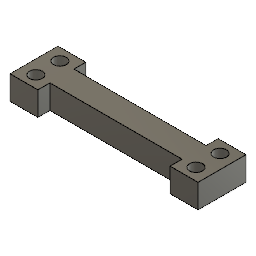
enclosure v64 (Autodesk Fusion 360 archive; units mm, degrees)
design "Load Cell"
Autodesk Fusion 360 part; units mm, degrees
sketch "Sketch1" plane through (0, 0, 0) normal (0, 1, 0) x (1, 0, 0)
  circle A0 centre (0, 0) radius 1.6
  line L0 (0, 0) -> (0, -6) construction
  circle A1 centre (0, -6) radius 1.6
  line L1 (0, -3) -> (40, -3) construction
  line L2 (-3.5, 3) -> (3.5, 3)
  line L3 (3.5, 3) -> (3.5, -9)
  line L4 (3.5, -9) -> (-3.5, -9)
  line L5 (-3.5, -9) -> (-3.5, 3)
  line L6 (20, -3) -> (20, -8.5486) construction
  circle A2 centre (40, 0) radius 1.6
  circle A3 centre (40, -6) radius 1.6
  line L7 (40, 0) -> (40, -6) construction
  line L8 (36.5, 3) -> (36.5, -9)
  line L9 (36.5, -9) -> (43.5, -9)
  line L10 (43.5, -9) -> (43.5, 3)
  line L11 (43.5, 3) -> (36.5, 3)
  line L12 (3.5, -0.0084) -> (36.5, -0.0084)
  line L13 (36.5, -0.0084) -> (36.5, -5.9916)
  line L14 (36.5, -5.9916) -> (3.5, -5.9916)
  line L15 (3.5, -5.9916) -> (3.5, -0.0084)
  point P0 (40, 0)
  point P1 (40, -3)
  dimension "d1" = 3.2
  dimension "d2" = 6
  dimension "d3" = 3.2
  dimension "d5" = 40
  dimension "d6" = 7
  dimension "d7" = 12
  constraint coincident A0.centre L0.start
  constraint vertical L0
  constraint coincident L0.end A1.centre
  constraint midpoint L0 L1.start
  constraint perpendicular L0 L1
  constraint horizontal L2
  constraint vertical L3
  constraint horizontal L4
  constraint vertical L5
  constraint symmetric L0 L3 L5
  constraint symmetric L1 L2 L4
  constraint midpoint L1 L6.start
  constraint perpendicular L1 L6
  constraint symmetric A0.centre L6 A2.centre
  constraint symmetric A0 L6 A2
  constraint symmetric A0.centre L6 P0
  constraint symmetric L0.end L6 A3.centre
  constraint symmetric A1 L6 A3
  constraint symmetric L1.start L6 P1
  constraint symmetric L2.start L6 L10.end
  constraint symmetric L2.end L6 L8.start
  constraint symmetric L3.end L6 L8.end
  constraint symmetric L4.end L6 L9.end
  constraint horizontal L12
  constraint vertical L13
  constraint horizontal L14
  constraint vertical L15
  constraint coincident L8 L13.end
  constraint coincident L3 L12.start
  constraint symmetric L1 L12 L14
  measures "d1" diameter of A0
  measures "d2" distance of A0.centre L0.end
  measures "d3" diameter of A1
  measures "d5" distance of L0 P1
  measures "d6" distance of L2.start L2.end
  measures "d7" distance of L2.start L4.end
extrude "Extrude1" add sketch "Sketch1" along normal blind 6

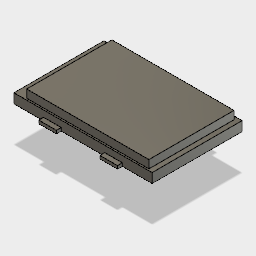
design "Display"
Autodesk Fusion 360 part; units mm, degrees
sketch "Sketch1" plane through (0, 0, 0) normal (0, 1, 0) x (1, 0, 0)
  line L0 (0, 0) -> (86, 0)
  line L1 (86, 0) -> (86, -56)
  line L2 (86, -56) -> (0, -56)
  line L3 (0, -56) -> (0, 0)
  line L4 (7, -2) -> (83, -2)
  line L5 (83, -2) -> (83, -55)
  line L6 (83, -55) -> (7, -55)
  line L7 (7, -55) -> (7, -2)
  line L8 (18.5, 3) -> (29.5, 3)
  line L9 (29.5, 3) -> (29.5, -59)
  line L10 (29.5, -59) -> (18.5, -59)
  line L11 (18.5, -59) -> (18.5, 3)
  line L12 (43, 0) -> (43, -72.5611) construction
  line L13 (86, -28) -> (0, -28) construction
  line L14 (67.5, 3) -> (56.5, 3)
  line L15 (56.5, 3) -> (56.5, -59)
  line L16 (67.5, -59) -> (67.5, 3)
  line L17 (56.5, -59) -> (67.5, -59)
  point P0 (43, 0)
  dimension "d9" = 86
  dimension "d10" = 56
  dimension "d11" = 76
  dimension "d12" = 53
  dimension "d13" = 7
  dimension "d14" = 2
  dimension "d18" = 62
  dimension "d19" = 11
  dimension "d20" = 13.5
  measures "d9" distance of L0.start L0.end
  measures "d10" distance of L0.start L2.end
  measures "d11" distance of L4.start L4.end
  measures "d12" distance of L4.start L6.end
  measures "d13" distance of L3 L7
  measures "d14" distance of L0 L4
  measures "d18" distance of L8.start L10.end
  measures "d19" distance of L8.start L8.end
  measures "d20" distance of L9 L12
extrude "Extrude1" add sketch "Sketch1" along normal blind 6 contours L0 L2 L3 L4 L6 L7 L11 | L0 L4 L9 L11 | L0 L4 L9 L15 | L4 L6 L7 L11 | L4 L6 L9 L11 | L2 L6 L9 L11 | L0 L4 L15 L16 | L4 L6 L9 L15 | L2 L6 L9 L15 | L0 L1 L2 L4 L5 L6 L16 | L4 L6 L15 L16 | L2 L6 L15 L16 | L4 L5 L6 L16 makes body 1
extrude "Extrude2" add sketch "Sketch1" along normal blind 11 separate body contours L4 L6 L7 L11 | L4 L6 L9 L11 | L4 L6 L9 L15 | L4 L6 L15 L16 | L4 L5 L6 L16 makes body 2
sketch "Sketch2" plane through (0, 0, 0) normal (0, 1, 0) x (1, 0, 0)
  line L0 (42, 0) -> (7, 0)
  line L1 (7, 0) -> (7, -6)
  line L2 (7, -6) -> (42, -6)
  line L3 (42, -6) -> (42, 0)
  line L4 (86, 0) -> (0, 0)
  line L5 (0, 0) -> (86, 0)
  line L6 (86, 0) -> (86, -56)
  line L7 (0, -56) -> (0, 0)
  dimension "d25" = 35
  dimension "d26" = 6
  dimension "d30" = 7
  measures "d25" distance of L0.start L0.end
  measures "d26" distance of L0.start L2.end
  measures "d30" distance of L1 L7
extrude "Extrude3" add sketch "Sketch2" against normal blind 22 bodies 1 2
extrude "Extrude4" add sketch "Sketch1" along normal blind 2 contours L0 L8 L9 L11 | L2 L9 L10 L11 | L0 L14 L15 L16 | L2 L15 L16 L17 bodies 1
equation "width = 85 mm"
equation "height = 55 mm"
equation "gap = 0.5 mm"
equation "visible_width = 76 mm"
equation "visible_height = 53 mm"
equation "visible_offset_x = 7 mm"
equation "visible_offset_y = 2 mm"
equation "thickness = 6 mm"
equation "d9 = width + 2 * gap"
equation "d10 = height + 2 * gap"
equation "d11 = visible_width"
equation "d12 = visible_height"
equation "d13 = visible_offset_x"
equation "d14 = visible_offset_y"
equation "tab_width = 10 mm"
equation "tab_height = 3 mm"
equation "tab_distance = 28 mm"
equation "d18 = height + 2 * tab_height + 2 * gap"
equation "d19 = tab_width + 2 * gap"
equation "d20 = tab_distance / 2 - gap"
equation "d21 = thickness"
equation "d23 = thickness + 5 mm"

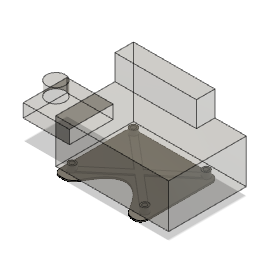
design "Electronics"
Autodesk Fusion 360 part; units mm, degrees
sketch "Sketch1" plane through (0, 0, 0) normal (0, 1, 0) x (1, 0, 0)
  line L0 (0, 0) -> (90, 0)
  line L1 (90, 0) -> (90, -62)
  line L2 (90, -62) -> (0, -62)
  line L3 (0, -62) -> (0, 0)
  line L4 (0, 0) -> (64.9649, 0)
  line L5 (64.9649, 0) -> (64.9649, -14.7819)
  line L6 (64.9649, -14.7819) -> (0, -14.7819)
  line L7 (0, -14.7819) -> (0, 0)
  dimension "d1" = 90
  dimension "d2" = 62
  constraint horizontal L0
  constraint vertical L1
  constraint horizontal L2
  constraint vertical L3
  constraint coincident L0.start L3.end
  constraint horizontal L4
  constraint vertical L5
  constraint horizontal L6
  constraint vertical L7
  measures "d1" distance of L0.start L0.end
  measures "d2" distance of L0.start L2.end
extrude "Extrude1" add sketch "Sketch1" along normal blind 35 makes body 1
extrude "Extrude2" add sketch "Sketch1" along normal blind 55 contours L0 L3 L4 L5 L6 L7 bodies 1
sketch "Sketch2" plane through (0, 0, 0) normal (-1, 0, 0) x (0, 0, 1)
  line L0 (0, 0) -> (62, 0)
  line L1 (62, 0) -> (62, 35)
  line L2 (62, 35) -> (14.7819, 35)
  line L3 (14.7819, 35) -> (14.7819, 55)
  line L4 (14.7819, 55) -> (0, 55)
  line L5 (0, 55) -> (0, 0)
  line L6 (51.1665, 9.6117) -> (16.2802, 9.6117)
  line L7 (16.2802, 9.6117) -> (16.2802, 20.2132)
  line L8 (16.2802, 20.2132) -> (51.1665, 20.2132)
  line L9 (51.1665, 20.2132) -> (51.1665, 9.6117)
  constraint horizontal L6
  constraint vertical L7
  constraint horizontal L8
  constraint vertical L9
extrude "Extrude3" add sketch "Sketch2" along normal blind 36.811 contours L6 L7 L8 L9 bodies 1
sketch "Sketch3" plane through (0, 20.2132, 0) normal (0, 1, 0) x (-1, 0, 0)
  line L0 (0, 51.1665) -> (0, 16.2802)
  line L1 (0, 16.2802) -> (36.811, 16.2802)
  line L2 (36.811, 16.2802) -> (36.811, 51.1665)
  line L3 (36.811, 51.1665) -> (0, 51.1665)
  circle A0 centre (28.2212, 33.7234) radius 7.477
  dimension "d9" = 14.9539
  measures "d9" diameter of A0
extrude "Extrude4" add sketch "Sketch3" along normal blind 11.214 contours A0 bodies 1
sketch "Sketch4" plane through (0, 0, 0) normal (0, -1, 0) x (1, 0, 0)
  line L0 (0, 62) -> (0, 0) construction
  line L1 (0, 0) -> (90, 0) construction
  line L2 (90, 0) -> (90, 62)
  line L3 (90, 62) -> (0, 62)
  circle A0 centre (4, 53) radius 3
  circle A1 centre (4, 53) radius 1.8
  line L4 (0, 62) -> (0, 0) construction
  circle A2 centre (62, 53) radius 3
  circle A3 centre (62, 53) radius 1.8
  circle A4 centre (4, 4) radius 3
  circle A5 centre (4, 4) radius 1.8
  circle A6 centre (62, 4) radius 3
  circle A7 centre (62, 4) radius 1.8
  line L5 (0, 0) -> (90, 0) construction
  line L6 (67.8445, 57) -> (67.8445, 5)
  line L7 (62.8445, 0) -> (2.8445, 0)
  line L8 (-2.1555, 5) -> (-2.1555, 57)
  spline S0 degree 2 poles (13.254, 57.5525) (31.8057, 20.1203) (54.2525, 58.0726) knots 0.04606 0.04606 0.04606 0.95394 0.95394 0.95394
  line L9 (6.0861, 62.3124) -> (6.0861, 9.7817) construction
  arc A8 (67.8445, 57) -> (62.8445, 62) centre (62.8445, 57) ccw
  arc A9 (2.8445, 62) -> (-2.1555, 57) centre (2.8445, 57) ccw
  line L10 (2.8445, 62) -> (6.0861, 62)
  line L11 (61.1382, 62) -> (62.8445, 62)
  line L12 (33.6122, 62) -> (55.9607, 62)
  arc A10 (13.254, 57.5525) -> (6.0861, 62) centre (6.0861, 54) ccw
  arc A11 (61.1382, 62) -> (54.2525, 58.0726) centre (61.1382, 54) ccw
  line L13 (13.254, 57.5525) -> (31.8057, 20.1203)
  line L14 (31.8057, 20.1203) -> (54.2525, 58.0726)
  line L15 (2.3866, 51.0903) -> (60.3866, 2.0903)
  arc A12 (60.3866, 2.0903) -> (63.6134, 5.9097) centre (62, 4) ccw
  line L16 (63.6134, 5.9097) -> (5.6134, 54.9097)
  arc A13 (5.6134, 54.9097) -> (2.3866, 51.0903) centre (4, 53) ccw
  line L17 (4, 53) -> (62, 4) construction
  line L18 (60.3866, 54.9097) -> (2.3866, 5.9097)
  arc A14 (2.3866, 5.9097) -> (5.6134, 2.0903) centre (4, 4) ccw
  line L19 (5.6134, 2.0903) -> (63.6134, 51.0903)
  arc A15 (63.6134, 51.0903) -> (60.3866, 54.9097) centre (62, 53) ccw
  line L20 (62, 53) -> (4, 4) construction
  arc A16 (62.8445, 0) -> (67.8445, 5) centre (62.8445, 5) ccw
  arc A17 (-2.1555, 5) -> (2.8445, 0) centre (2.8445, 5) ccw
  line L21 (-4.6829, 40.4604) -> (70.3171, 40.4604)
  line L22 (70.3171, 40.4604) -> (70.3171, 0)
  line L23 (70.3171, 0) -> (-4.6829, 0)
  line L24 (-4.6829, 0) -> (-4.6829, 40.4604)
  dimension "d12" = 6
  dimension "d13" = 3.6
  dimension "d23" = 4
  dimension "d26" = 58
  dimension "d27" = -49
  dimension "d28" = 4
  dimension "d29" = 70
  dimension "d30" = 5
  dimension "d31" = 5
  dimension "d32" = 8
  dimension "d33" = 8
  dimension "d44" = 5
  dimension "d45" = 5
  dimension "d46" = 5
  dimension "d47" = 5
  dimension "d48" = 75
  constraint concentric A0 A1
  constraint horizontal L10
  constraint vertical L6
  constraint horizontal L7
  constraint vertical L8
  constraint coincident L12.end L10
  constraint perpendicular L9 L10
  constraint tangent A8 L10
  constraint tangent L6 A8
  constraint tangent L8 A9
  constraint tangent A9 L10
  constraint coincident L9 L10.end
  constraint tangent S0 A10
  constraint tangent L10 A10
  constraint coincident L12.end L11
  constraint tangent S0 A11
  constraint tangent L11 A11
  constraint tangent L15 A12
  constraint tangent A12 L16
  constraint parallel L15 L16
  constraint tangent L16 A13
  constraint tangent L15 A13
  constraint coincident A6.centre A7.centre
  constraint coincident A0.centre A1.centre
  constraint tangent L18 A14
  constraint tangent A14 L19
  constraint parallel L18 L19
  constraint tangent L19 A15
  constraint tangent L18 A15
  constraint coincident A4.centre A5.centre
  constraint coincident A2.centre A3.centre
  constraint tangent L6 A16
  constraint tangent L7 A16
  constraint tangent L8 A17
  constraint tangent L7 A17
  constraint horizontal L21
  constraint vertical L22
  constraint horizontal L23
  constraint vertical L24
  constraint coincident L5 L22.end
  measures "d12" diameter of A0
  measures "d13" diameter of A1
  measures "d23" distance of A0.centre L4
  measures "d28" distance of A4.centre L5
  measures "d29" distance of L6 L8
  measures "d30" radius of A8
  measures "d31" radius of A9
  measures "d32" radius of A10
  measures "d33" radius of A11
  measures "d44" diameter of A12
  measures "d45" diameter of A14
  measures "d46" radius of A16
  measures "d47" radius of A17
  measures "d48" distance of L22 L24
extrude "Extrude5" add sketch "Sketch4" along normal blind 1.25 from surface at 5 separate body contours L3 A2 L6 A8 L11 A11 L14 L18 L19 L21 | S0 L14 L18 L21 | A4 A6 L6 L7 L8 L13 L14 L15 L16 L18 L19 A16 A17 L21 L23 | S0 L16 L18 L21 | A2 L14 L18 L19 L21 | L14 L18 L21 | L14 L16 L19 L21 | L3 A0 L8 A9 L10 A10 L13 L15 L16 L21 | S0 L13 L16 L21 | L14 L16 L18 L21 | A2 L18 L19 A15 | A2 L18 L19 A15 | L14 L16 L19 | A6 L14 L15 L16 L19 | L13 L16 L21 | L13 L15 L16 L18 L21 | L14 L15 L16 L18 L19 | A6 L15 A12 L16 | A6 L15 A12 L16 | L14 L15 L19 | A0 L13 L15 L16 L21 | L13 L15 L21 | L13 L15 L18 | L13 L15 L18 L19 | L13 L14 L15 L19 | A0 L15 L16 A13 | A0 L15 L16 A13 | A4 L13 L18 L19 | A4 L18 A14 L19 | A4 L18 A14 L19 | A1 | A3 | A5 | A7 makes body 2
extrude "Extrude6" add sketch "Sketch4" along normal blind 5 contours A2 L18 L19 A15 | A2 L18 L19 A15 | A6 L15 A12 L16 | A6 L15 A12 L16 | A0 L15 L16 A13 | A0 L15 L16 A13 | A4 L18 A14 L19 | A4 L18 A14 L19 bodies 2
extrude "Extrude7" add sketch "Sketch4" against normal blind 1 from surface at 5 contours A2 L14 L18 L19 L21 | L14 L18 L21 | L14 L16 L19 L21 | L14 L16 L18 L21 | A2 L18 L19 A15 | L14 L16 L19 | A6 L14 L15 L16 L19 | L13 L16 L21 | L13 L15 L16 L18 L21 | L14 L15 L16 L18 L19 | A6 L15 A12 L16 | L14 L15 L19 | A0 L13 L15 L16 L21 | L13 L15 L21 | L13 L15 L18 L19 | A0 L15 L16 A13 | A4 L13 L18 L19 | A4 L18 A14 L19 picked at (62.8725, 50.8116) picked at (62.8725, 6.1884) picked at (3.1275, 50.8116) picked at (3.1275, 6.1884) bodies 2
extrude "Extrude8" add sketch "Sketch4" against normal blind 1.5 from surface at 6.25 separate body contours L6 A16 L21 L22 L23 | A4 A6 L6 L7 L8 L13 L14 L15 L16 L18 L19 A16 A17 L21 L23 | S0 L16 L18 L21 | S0 L21 | L14 L16 L19 L21 | L14 L16 L18 L21 | L14 L16 L19 | A6 L14 L15 L16 L19 | L13 L15 L16 L18 L21 | L14 L15 L16 L18 L19 | L8 A17 L21 L23 L24 | A6 L15 A12 L16 | A6 L15 A12 L16 | L14 L15 L19 | L13 L15 L21 | L13 L15 L18 | L13 L15 L18 L19 | L13 L14 L15 L19 | A4 L13 L18 L19 | A4 L18 A14 L19 | A4 L18 A14 L19 | A5 | A7 makes body 3
hidden bodies 3
named bodies: "Dummy", "RaspiHolder", "RaspiHolderNegative"

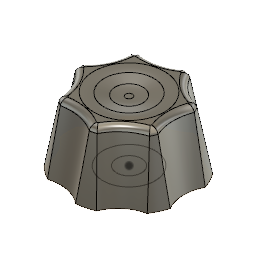
design "knob"
Autodesk Fusion 360 part; units mm, degrees
sketch "Sketch1" plane through (0, 0, 0) normal (0, 1, 0) x (1, 0, 0)
  circle A0 centre (0, 0) radius 15
  circle A1 centre (13.6368, 17.9706) radius 9.3906
  circle A2 centre (-5.5475, 21.8662) radius 9.3906
  circle A3 centre (-20.5545, 9.2961) radius 9.3906
  circle A4 centre (-20.0835, -10.2741) radius 9.3906
  circle A5 centre (-4.4892, -22.1077) radius 9.3906
  circle A6 centre (14.4855, -17.2938) radius 9.3906
  circle A7 centre (22.5524, 0.5428) radius 9.3906
  dimension "d1" = 30
  dimension "d3" = 360
  constraint coincident A0.centre origin
  measures "d1" diameter of A0
extrude "Extrude1" add sketch "Sketch1" along normal blind 16 draft -10 contours A0 A1 A2 A3 A4 A5 A6 A7
fillet "Fillet1" radius 1.5 14 edges at (6.6441, 16, 7.9321) (2.9949, 16, 11.8048) (-2.0591, 16, 10.1401) (-7.362, 16, 9.7017) (-9.2117, 16, 4.7124) (-12.1752, 16, 0.293) (-9.4277, 16, -4.2638) (-7.8202, 16, -9.3363) (-2.5445, 16, -10.0293) (2.4236, 16, -11.9352) (6.2548, 16, -8.2426) (10.8424, 16, -5.5466) (10.3441, 16, -0.249) (11.0967, 16, 5.0186)
sketch "Sketch2" plane through (0, 16, 0) normal (0, 1, 0) x (-1, 0, 0)
  arc A0 (6.9002, -8.4638) -> (-2.0308, -10.7296) centre (5.5475, -21.8662) ccw
  arc A1 (6.9002, -8.4638) -> (7.1226, -8.2776) centre (0, 0) ccw
  arc A2 (10.9195, 0.1177) -> (7.1226, -8.2776) centre (20.5545, -9.2961) ccw
  arc A3 (10.9195, 0.1177) -> (10.9125, 0.4077) centre (0, 0) ccw
  arc A4 (6.7161, 8.6106) -> (10.9125, 0.4077) centre (20.0835, 10.2741) ccw
  arc A5 (6.7161, 8.6106) -> (6.4851, 8.7859) centre (0, 0) ccw
  arc A6 (-2.5446, 10.6195) -> (6.4851, 8.7859) centre (4.4892, 22.1077) ccw
  arc A7 (-2.5446, 10.6195) -> (-2.8257, 10.5482) centre (0, 0) ccw
  arc A8 (-9.8892, 4.6317) -> (-2.8257, 10.5482) centre (-14.4855, 17.2938) ccw
  arc A9 (-9.8892, 4.6317) -> (-10.0087, 4.3675) centre (0, 0) ccw
  arc A10 (-9.787, -4.8439) -> (-10.0087, 4.3675) centre (-22.5524, -0.5428) ccw
  arc A11 (-9.787, -4.8439) -> (-9.6549, -5.1021) centre (0, 0) ccw
  arc A12 (-2.315, -10.6719) -> (-9.6549, -5.1021) centre (-13.6368, -17.9706) ccw
  arc A13 (-2.315, -10.6719) -> (-2.0308, -10.7296) centre (0, 0) ccw
  circle A14 centre (0, 0) radius 7.5
  dimension "d9" = 15
  constraint concentric A1 A14
  measures "d9" diameter of A14
extrude "Extrude2" cut sketch "Sketch2" against normal blind 0.942 draft -80 contours A14
fillet "Fillet2" radius 15 2 edges at (6.9925, 16, 2.7121) (2.0116, 15.058, -0.7802)
sketch "Sketch3" plane through (0, 0, 0) normal (0, -1, 0) x (1, 0, 0)
  arc A0 (5.7471, 13.8554) -> (1.5532, 14.9194) centre (0, 0) ccw
  arc A1 (-7.2493, 13.1319) -> (1.5532, 14.9194) centre (-4.4892, 22.1077) ccw
  arc A2 (-7.2493, 13.1319) -> (-10.696, 10.5164) centre (0, 0) ccw
  arc A3 (-14.7868, 2.5199) -> (-10.696, 10.5164) centre (-20.0835, 10.2741) ccw
  arc A4 (-14.7868, 2.5199) -> (-14.8909, -1.8056) centre (0, 0) ccw
  arc A5 (-11.1895, -9.9897) -> (-14.8909, -1.8056) centre (-20.5545, -9.2961) ccw
  arc A6 (-11.1895, -9.9897) -> (-7.8727, -12.768) centre (0, 0) ccw
  arc A7 (0.8337, -14.9768) -> (-7.8727, -12.768) centre (-5.5475, -21.8662) ccw
  arc A8 (0.8337, -14.9768) -> (5.0739, -14.1158) centre (0, 0) ccw
  arc A9 (12.2291, -8.6861) -> (5.0739, -14.1158) centre (13.6368, -17.9706) ccw
  arc A10 (12.2291, -8.6861) -> (14.1997, -4.8341) centre (0, 0) ccw
  arc A11 (14.4158, 4.1455) -> (14.1997, -4.8341) centre (22.5524, -0.5428) ccw
  arc A12 (14.4158, 4.1455) -> (12.6328, 8.0877) centre (0, 0) ccw
  arc A13 (5.7471, 13.8554) -> (12.6328, 8.0877) centre (14.4855, 17.2938) ccw
  circle A14 centre (0, 0) radius 6.5
  circle A15 centre (0, 0) radius 3.1
  dimension "d11" = 6.2
  dimension "d14" = 13
  constraint concentric A0 A14
  constraint concentric A14 A15
  measures "d11" diameter of A15
  measures "d14" diameter of A14
extrude "Extrude3" cut sketch "Sketch3" against normal blind 4.0266 draft -40 contours A14 | A15
extrude "Extrude4" cut sketch "Sketch3" against normal blind 13 contours A15
named bodies: "Knob"
